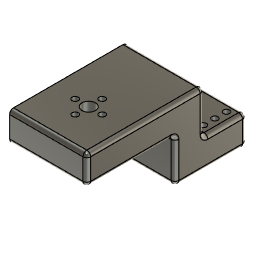
tetris (Autodesk Fusion 360 design; units mm, degrees)
Autodesk Fusion 360 part; units mm, degrees
sketch "Sketch1" plane through (0, 0, 0) normal (1, 0, 0) x (0, 1, 0)
  line L0 (0, 0) -> (0, -15)
  line L1 (0, -15) -> (30, -15)
  line L2 (30, -15) -> (45.75, -15)
  line L3 (60.75, -15) -> (60.75, -22.5)
  line L4 (60.75, -37.5) -> (82.75, -37.5)
  line L5 (82.75, -37.5) -> (82.75, -22.5)
  line L6 (60.75, 0) -> (0, 0)
  line L7 (45.75, -15) -> (45.75, -37.5)
  line L8 (45.75, -37.5) -> (60.75, -37.5)
  line L9 (60.75, 0) -> (60.75, -15)
  line L10 (60.75, -22.5) -> (82.75, -22.5)
  dimension "d1" = 15
  dimension "d2" = 30
  dimension "d3" = 30.75
  dimension "d4" = 22.5
  dimension "d5" = 22
  dimension "d6" = 15
  dimension "d8" = 15
  dimension "d9" = 15
  constraint coincident L0.start L6.end
  constraint vertical L0
  constraint perpendicular L0 L1
  constraint parallel L1 L2
  constraint perpendicular L2 L3
  constraint perpendicular L3 L4
  constraint perpendicular L1 L5
  constraint perpendicular L0 L6
  constraint perpendicular L4 L7
  constraint perpendicular L3 L8
  constraint perpendicular L2 L9
  measures "d1" distance of L0.start L0.end
  measures "d2" distance of L0.end L1.end
  measures "d3" distance of L1.end L3.start
  measures "d4" distance of L3.start L4.start
  measures "d5" distance of L4.start L4.end
  measures "d6" distance of L4.end L5.end
  measures "d8" distance of L3.start L2.end
  measures "d9" distance of L4.start L3.end
extrude "Extrude1" add sketch "Sketch1" along normal blind 40
sketch "Sketch2" plane through (0, 0, -22.5) normal (0, 0, 1) x (-1, 0, 0)
  line L0 (0, -82.75) -> (0, -60.75)
  line L1 (0, -60.75) -> (-40, -60.75)
  line L2 (-40, -60.75) -> (-40, -82.75)
  line L3 (-40, -82.75) -> (0, -82.75)
  line L4 (-40, -82.75) -> (-34.9, -82.75) construction
  line L5 (-20, -82.75) -> (-20, -60.75) construction
  line L6 (-20, -77.95) -> (-5.5, -77.95) construction
  circle A0 centre (-5.5, -77.95) radius 1.6
  circle A1 centre (-5.5, -71.95) radius 1.6
  circle A2 centre (-5.5, -65.95) radius 1.6
  circle A3 centre (-34.5, -77.95) radius 1.6
  circle A4 centre (-34.5, -71.95) radius 1.6
  circle A5 centre (-34.5, -65.95) radius 1.6
  dimension "d40" = 3.2
  dimension "d41" = 3.2
  dimension "d42" = 3.2
  constraint coincident L2.end L3.start
  constraint coincident L3 L4.end
  constraint midpoint L3 L5.start
  constraint midpoint L1 L5.end
  constraint coincident L5 L6.start
  constraint coincident L6.end A0.centre
  constraint symmetric L5 A0 A3
  constraint symmetric L5 A1 A4
  constraint symmetric L5 A2 A5
  measures "d40" diameter of A0
  measures "d41" diameter of A1
  measures "d42" diameter of A2
fillet "Fillet1" radius 2 8 edges at (20, 0, 0) (20, 0, -15) (20, 60.75, 0) (20, 60.75, -22.5) (20, 82.75, -22.5) (20, 82.75, -37.5) (20, 45.75, -37.5) (20, 45.75, -15)
fillet "Fillet2" radius 2 16 edges at (40, 0.5858, -0.5858) (40, 0, -7.5) (40, 0.5858, -14.4142) (40, 22.875, -15) (40, 45.1642, -15.5858) (40, 45.75, -26.25) (40, 46.3358, -36.9142) (40, 64.25, -37.5) (40, 82.1642, -36.9142) (40, 82.75, -30) (40, 82.1642, -23.0858) (40, 71.75, -22.5) (40, 61.3358, -21.9142) (40, 60.75, -11.25) (40, 60.1642, -0.5858) (40, 30.375, 0)
sketch "Sketch3" plane through (0, 0, 0) normal (0, 0, 1) x (-1, 0, 0)
  line L0 (-38, -2) -> (-38, -58.75)
  line L1 (-38, -58.75) -> (0, -58.75)
  line L2 (0, -58.75) -> (0, -2)
  line L3 (0, -2) -> (-38, -2)
  circle A0 centre (-19, -11.5) radius 0.8
  line L4 (-19, -22) -> (-19, -14.5) construction
  circle A1 centre (-30.6913, -28.75) radius 0.8
  circle A2 centre (-12.5048, -25.75) radius 0.8
  circle A3 centre (-35.5, -22) radius 0.8
  circle A4 centre (-19, -5.5) radius 0.8
  circle A5 centre (-33.2894, -13.75) radius 0.8
  circle A6 centre (-19, -32.5) radius 0.8
  circle A7 centre (-28.0933, -27.25) radius 0.8
  circle A8 centre (-12.5048, -18.25) radius 0.8
  circle A9 centre (-32.5, -22) radius 0.8
  line L5 (-19, 19.2574) -> (-19, -41.0839) construction
  circle A10 centre (-25.4952, -18.25) radius 0.8
  circle A11 centre (-2.5, -22) radius 0.8
  line L6 (-19, -22) -> (-19, -5.5) construction
  circle A12 centre (-9.9067, -16.75) radius 0.8
  circle A13 centre (-30.6913, -15.25) radius 0.8
  circle A14 centre (-8.5, -22) radius 0.8
  circle A15 centre (-7.3087, -28.75) radius 0.8
  circle A16 centre (-28.0933, -16.75) radius 0.8
  circle A17 centre (-19, -38.5) radius 0.8
  line L7 (-19, -22) -> (-19, -8.5) construction
  circle A18 centre (-19, -29.5) radius 0.8
  line L8 (-19, -22) -> (-19, -11.5) construction
  circle A19 centre (-5.5, -22) radius 0.8
  circle A20 centre (-19, -35.5) radius 0.8
  circle A21 centre (-11.5, -22) radius 0.8
  circle A22 centre (-29.5, -22) radius 0.8
  circle A23 centre (-19, -22) radius 19
  circle A24 centre (-4.7106, -30.25) radius 0.8
  circle A25 centre (-33.2894, -30.25) radius 0.8
  circle A26 centre (-19, -14.5) radius 0.8
  circle A27 centre (-25.4952, -25.75) radius 0.8
  circle A28 centre (-9.9067, -27.25) radius 0.8
  circle A29 centre (-26.5, -22) radius 0.8
  circle A30 centre (-7.3087, -15.25) radius 0.8
  circle A31 centre (-4.7106, -13.75) radius 0.8
  circle A32 centre (-19, -8.5) radius 0.8
  line L9 (0, -2) -> (-19, -2) construction
  line L10 (-19, -2) -> (-19, -22) construction
  point P0 (-19, -22)
  dimension "d25" = 360
  dimension "d27" = 90
  dimension "d28" = 38
  dimension "d29" = 7.5
  dimension "d30" = 1.6
  dimension "d31" = 10.5
  dimension "d32" = 1.6
  dimension "d33" = 13.5
  dimension "d34" = 1.6
  dimension "d35" = 16.5
  dimension "d36" = 1.6
  dimension "d37" = 20
  constraint coincident P0 L4.start
  constraint vertical L5
  constraint coincident L4.end L5
  constraint parallel L4 L5
  constraint coincident L4.end A26.centre
  constraint coincident A0.centre L5
  constraint coincident A0.centre L8.end
  constraint coincident L7.end L5
  constraint coincident L7.end A32.centre
  constraint coincident A4.centre L5
  constraint coincident A4.centre L6.end
  constraint symmetric L5 A21 A29
  constraint symmetric L5 A14 A22
  constraint symmetric A9 L5 A19
  constraint symmetric A3 L5 A11
  constraint coincident L2.end L3.start
  constraint midpoint L3 L9.end
  constraint perpendicular L9 L10
  measures "d28" diameter of A23
  measures "d29" distance of L4.end P0
  measures "d30" diameter of A26
  measures "d31" distance of A0.centre P0
  measures "d32" diameter of A0
  measures "d33" distance of L7.end P0
  measures "d34" diameter of A32
  measures "d35" distance of P0 A4.centre
  measures "d36" diameter of A4
  measures "d37" distance of L9.end P0
extrude "Extrude4" cut sketch "Sketch2" against normal through all contours A0 | A1 | A2 | A3 | A4 | A5
sketch "Sketch4" plane through (0, 0, 0) normal (0, 0, 1) x (-1, 0, 0)
  line L0 (-38, -2) -> (-38, -58.75)
  line L1 (-38, -58.75) -> (0, -58.75)
  line L2 (0, -58.75) -> (0, -2)
  line L3 (0, -2) -> (-38, -2)
  line L4 (-19, -2) -> (-19, -22) construction
  circle A0 centre (-19, -22) radius 19
  line L5 (-19, -22) -> (-19, -29) construction
  circle A1 centre (-19, -29) radius 1.6
  circle A2 centre (-12, -22) radius 1.6
  circle A3 centre (-19, -15) radius 1.6
  circle A4 centre (-26, -22) radius 1.6
  circle A5 centre (-19, -22) radius 3.5
  dimension "d44" = 20
  dimension "d45" = 38
  dimension "d46" = 7
  dimension "d47" = 3.2
  dimension "d49" = 360
  dimension "d50" = 7
  constraint midpoint L3 L4.start
  constraint perpendicular L3 L4
  constraint coincident L4.end A0.centre
  constraint parallel L4 L5
  constraint coincident L5.end A1.centre
  constraint concentric A0 A5
  measures "d44" distance of L4.start L4.end
  measures "d45" diameter of A0
  measures "d46" distance of L4.end L5.end
  measures "d47" diameter of A1
  measures "d50" diameter of A5
extrude "Extrude5" cut sketch "Sketch4" against normal through all contours A1 | A2 | A3 | A4 | A5
equation "d29 = ( 15 / 2 ) * 1 mm"
equation "d31 = ( 21 / 2 ) * 1 mm"
equation "d33 = ( 27 / 2 ) * 1 mm"
equation "d35 = ( 33 / 2 ) * 1 mm"
equation "d46 = ( 14 / 2 ) * 1 mm"
